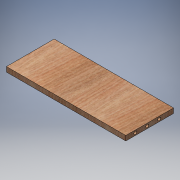
# Autodesk Inventor part: Steckwand
Saved by Autodesk Inventor 2016 SP2 (Build 200236200, 236)
## iProperties
Category: -50
Company: USK - Karl Utz Sondermaschinen GmbH
Created: 2018-05-28
Part Number: Steckwand
Material: Spanplatte
Description: 1
Document SubType Name: Modeling
Designer: Granz
Manufacturer: Standard
Standards Organization: Custom
Mass: 1016.7 g
Surface Area: 1487.87 cm^2
Volume: 1016.7 cm^3
Density: 1 g/cm^3
Appearance: Birke - natur- poliert
Author: Granz
Autodesk Inventor part; units mm, degrees
ref_plane "YZ Ebene" through (0, 0, 0) normal (1, 0, 0) x (0, 1, 0)
ref_plane "XZ Ebene" through (0, 0, 0) normal (0, 1, 0) x (-1, 0, 0)
ref_plane "XY Ebene" through (0, 0, 0) normal (0, 0, 1) x (1, 0, 0)
sketch "Langloch" plane through (0, 0, 0) normal (0, 0, 1) x (1, 0, 0)
  line L0 (-9.675, 3.175) -> (9.675, 3.175)
  line L1 (9.675, -3.175) -> (-9.675, -3.175)
  arc A0 (-9.675, 3.175) -> (-9.675, -3.175) centre (-9.675, 0) ccw
  arc A1 (9.675, -3.175) -> (9.675, 3.175) centre (9.675, 0) ccw
  line L2 (-9.675, 0) -> (9.675, 0) construction
  point P0 (0, 0)
  point P1 (0, 0)
  dimension "d6" = 6.35
  dimension "d7" = 19.35
  measures "d6" distance between parallel lines of L1 L0
  measures "d7" distance of L0.start L0.end
sketch "Skizze1" plane through (0, 0, 0) normal (0, 0, 1) x (1, 0, 0)
  line L0 (0, -112) -> (0, 112) projected
  line L1 (-280, 0) -> (280, 0) projected
  line L2 (-200, 80) -> (200, 80)
  line L3 (200, 80) -> (200, -80)
  line L4 (200, -80) -> (-200, -80)
  line L5 (-200, -80) -> (-200, 80)
  point P0 (0, 0)
  dimension "d10" = 160
  dimension "d11" = 80
  dimension "d12" = 400
  dimension "d13" = 200
  constraints: 8 end point, 2 parallel, 1 horizontal, 1 perpendicular
  measures "d10" distance of L2.end L3.end
  measures "d11" distance between parallel lines of L1 L2
  measures "d12" distance of L2.start L2.end
  measures "d13" distance between parallel lines of L0 L3
extrude "Extrusion4" add sketch "Skizze1" along normal blind 16
sketch "Skizze3" plane through (200, -80, 0) normal (1, 0, 0) x (0, 0, -1)
  line L0 (0, 160) -> (0, 0) projected
  line L1 (0, 160) -> (-16, 160) projected
  line L2 (-16, 0) -> (-16, 160) projected
  line L3 (0, 0) -> (-16, 0) projected
  point P0 (0, 80)
  point P1 (-8, 112)
  point P2 (-8, 72)
  point P3 (-8, 32)
  point P4 (-8, 160)
  dimension "d18" = 48
  dimension "d19" = 40
  dimension "d20" = 40
  constraints: 3 vertical alignment, 1 midpoint
  measures "d18" distance from line of point (-8, 112) L1
  measures "d19" distance of point (-8, 72) point (-8, 112)
  measures "d20" distance of point (-8, 32) point (-8, 72)
hole "Bohrung1" at (200, 32, 8) at (200, -8, 8) at (200, -48, 8) direction (-1, 0, 0) diameter 10 depth 30 tip angle 118
equation "\"d11\" = 0.5 * d10"
equation "\"d13\" = 0.5 * d12"
